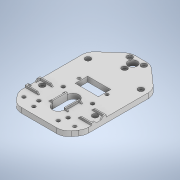
# Autodesk Inventor part: chassis
Saved by Autodesk Inventor 2020 (Build 240168000, 168)
## iProperties
Created: 2020-11-03
Part Number: chassis
Material: Generic
Document SubType Name: Modeling
Designer: alnwlsn
Density: 1 g/cm^3
Appearance: Default
Author: alnwlsn
Autodesk Inventor part; units mm, degrees
ref_plane "YZ Plane" through (0, 0, 0) normal (1, 0, 0) x (0, 1, 0)
ref_plane "XZ Plane" through (0, 0, 0) normal (0, 1, 0) x (-1, 0, 0)
sketch "Sketch1" plane through (0, 0, 0) normal (0, 1, 0) x (-1, 0, 0)
  line L0 (0, 0) -> (0, -80)
  line L1 (22.5, -100) -> (42.5, -100)
  line L2 (42.5, -100) -> (65, -80)
  line L3 (65, -80) -> (65, 0)
  line L4 (65, 0) -> (0, 0)
  line L5 (65, -80) -> (0, -80) construction
  line L6 (0, -80) -> (22.5, -100)
  line L7 (32.5, -100) -> (32.5, -80) construction
  line L8 (56, 0) -> (65, -12)
  line L9 (9, 0) -> (0, -12)
  dimension "d0" = 65
  dimension "d1" = 80
  dimension "d2" = 20
  dimension "d3" = 20
  dimension "d66" = 9
  dimension "d67" = 9
  dimension "d68" = 12
  dimension "d69" = 12
  constraints: 20 end point, 4 point on line, 3 perpendicular, 2 midpoint, 2 vertical, 1 parallel
  measures "d0" distance of L3.end L0.start
  measures "d1" distance of L2.end L3.end
  measures "d2" distance between parallel lines of L1 L5
  measures "d3" distance of L1.start L1.end
  measures "d66" distance of L3.end L8.start
  measures "d67" distance of L0.start L9.start
  measures "d68" distance of L0.start L9.end
  measures "d69" distance of L3.end L8.end
extrude "Extrusion1" add sketch "Sketch1" along normal blind 5 contours L9 L4 L8 L3 L2 L1 L6 L0
sketch "Sketch2" plane through (0, 5, 0) normal (0, 1, 0) x (1, 0, 0)
  line L0 (-1.2, 20) -> (-25.6, 20)
  line L1 (-25.6, 20) -> (-25.6, 32.2)
  line L2 (-25.6, 32.2) -> (-1.2, 32.2)
  line L3 (-1.2, 32.2) -> (-1.2, 20)
  line L4 (0, 33.4) -> (-26.8, 33.4)
  line L5 (-26.8, 33.4) -> (-26.8, 18.8)
  line L6 (-26.8, 18.8) -> (0, 18.8)
  line L7 (0, 18.8) -> (0, 33.4)
  line L8 (-56, 0) -> (0, 0) projected
  line L9 (-1.2, 23.8) -> (0, 23.8)
  line L10 (-1.2, 28.4) -> (0, 28.4)
  line L11 (0, 0) -> (0, 80) projected
  line L12 (-23.1, 18.8) -> (-23.1, 33.4)
  line L13 (-13.1, 18.8) -> (-13.1, 33.4)
  point P0 (-65, 0)
  point P1 (0, 28.4)
  point P2 (-13.1, 32.2)
  point P3 (-13.1, 20)
  point P4 (-23.1, 32.2)
  point P5 (-23.1, 20)
  dimension "d6" = 1.2
  dimension "d7" = 12.2
  dimension "d8" = 24.4
  dimension "d9" = 20
  dimension "d12" = 5
  dimension "d13" = 5
  dimension "d17" = 10
  dimension "d19" = 2.5
  constraints: 24 end point, 9 point on line, 6 perpendicular, 4 parallel, 1 horizontal, 3 other
  measures "d6" distance between parallel lines of L4 L2
  measures "d7" distance between parallel lines of L2 L0
  measures "d8" distance between parallel lines of L1 L3
  measures "d9" distance between parallel lines of L8 L0
  measures "d12" distance between parallel lines of L4 L10
  measures "d13" distance between parallel lines of L9 L6
  measures "d17" distance between parallel lines of L13 L12
  measures "d19" distance between parallel lines of L1 L12
extrude "Extrusion2" add sketch "Sketch2" along normal blind 2 contours L3 L9 L7 L6 L13 L0 | L12 L6 L5 L4 L2 L1 L0 | L13 L4 L7 L10 L3 L2
chamfer "Chamfer1" distance 2 angle 45 6 edges at (-0.6, 7, -23.8) (-0.6, 7, -28.4) (-13.1, 7, -19.4) (-23.1, 7, -19.4) (-23.1, 7, -32.8) (-13.1, 7, -32.8)
ref_plane "Work Plane1" through (-32.5, 0, 0) normal (1, 0, 0) x (0, 0, -1)
sketch "Sketch3" plane through (0, 5, 0) normal (0, 1, 0) x (1, 0, 0)
  line L0 (-25.1, 18.8) -> (-23.1, 18.8) projected
  line L1 (-13.1, 33.4) -> (0, 33.4) projected
  line L2 (-23.1, 18.8) -> (-13.1, 33.4) construction
  line L3 (-18.1, 26.1) -> (-18.1, 38.1) construction
  line L4 (-18.1, 26.1) -> (-18.1, 14.1) construction
  circle A0 centre (-18.1, 14.1) radius 1.7
  circle A1 centre (-18.1, 38.1) radius 1.7
  point P0 (0, 0)
  dimension "d20" = 24
  dimension "d21" = 3.4
  constraints: 6 end point, 2 centre point, 2 coincident, 1 collinear, 1 equal radius, 1 midpoint, 1 point on line, 1 vertical
  measures "d20" distance of L4.end L3.end
  measures "d21" diameter of A1
extrude "Extrusion3" cut sketch "Sketch3" against normal through all
mirror "Mirror1" about plane through (-32.5, 0, 0) normal (1, 0, 0) of "Extrusion2", "Extrusion3", "Chamfer1"
sketch "Sketch4" plane through (0, 0, 0) normal (0, -1, 0) x (1, 0, 0)
  line L0 (-22.5, -100) -> (-42.5, -100) projected
  line L1 (-32.5, -100) -> (-32.5, -92) construction
  circle A0 centre (-32.5, -92) radius 4.5
  line L2 (-42.2859, -97.6499) -> (-22.7141, -97.6499) construction
  line L3 (-42.2859, -97.6499) -> (-32.5, -80.7002) construction
  line L4 (-32.5, -80.7002) -> (-22.7141, -97.6499) construction
  line L5 (-37.3929, -89.1751) -> (-22.7141, -97.6499) construction
  circle A1 centre (-32.5, -84.0002) radius 1.65
  circle A2 centre (-25.572, -95.9999) radius 1.65
  circle A3 centre (-39.428, -95.9999) radius 1.65
  point P0 (0, 0)
  point P1 (-32.5, -97.6499)
  dimension "d24" = 9
  dimension "d25" = 13.856
  dimension "d26" = 3.3
  dimension "d27" = 8
  constraints: 10 end point, 6 tangent, 4 centre point, 3 midpoint, 2 equal length, 2 equal radius, 2 point on line, 1 coincident, 1 horizontal, 1 vertical
  measures "d24" diameter of A0
  measures "d25" distance of A2.centre A3.centre
  measures "d26" diameter of A2
  measures "d27" distance of L1.start L1.end
extrude "Extrusion4" cut sketch "Sketch4" against normal through all
sketch "Sketch5" plane through (0, 0, 0) normal (0, -1, 0) x (1, 0, 0)
  line L0 (-65, -80) -> (-65, -33.4) projected
  line L1 (-65, -53) -> (0, -53) construction
  line L2 (-56, 0) -> (0, 0) projected
  line L3 (-43.85, -46.9) -> (-21.15, -46.9)
  line L4 (-21.15, -46.9) -> (-21.15, -59.1)
  line L5 (-21.15, -59.1) -> (-43.85, -59.1)
  line L6 (-43.85, -59.1) -> (-43.85, -46.9)
  line L7 (-43.85, -46.9) -> (-21.15, -59.1) construction
  line L8 (-21.15, -46.9) -> (-43.85, -59.1) construction
  line L9 (0, 0) -> (0, -80) projected
  circle A0 centre (-46.25, -53) radius 1.5
  circle A1 centre (-18.75, -53) radius 1.5
  point P0 (-65, 0)
  point P1 (-32.5, -53)
  dimension "d30" = 53
  dimension "d31" = 22.7
  dimension "d32" = 12.2
  dimension "d33" = 13.75
  dimension "d34" = 13.75
  dimension "d35" = 3
  constraints: 14 end point, 4 point on line, 3 midpoint, 2 centre point, 2 horizontal, 2 parallel, 1 equal radius, 1 perpendicular
  measures "d30" distance between parallel lines of L1 L2
  measures "d31" distance between parallel lines of L4 L6
  measures "d32" distance between parallel lines of L3 L5
  measures "d33" distance of point (-32.5, -53) A1.centre
  measures "d34" distance of A0.centre point (-32.5, -53)
  measures "d35" diameter of A1
extrude "Extrusion5" cut sketch "Sketch5" against normal through all
sketch "Sketch6" plane through (0, 5, 0) normal (0, 1, 0) x (1, 0, 0)
  line L0 (-44.5, 6.75) -> (-20.5, 6.75) construction
  circle A0 centre (-44.5, 6.75) radius 1.65
  circle A1 centre (-20.5, 6.75) radius 1.65
  line L1 (-32.5, 6.75) -> (-32.5, 0) construction
  line L2 (-56, 0) -> (-9, 0) projected
  point P0 (-65, 0)
  dimension "d38" = 3.3
  dimension "d40" = 24
  constraints: 4 end point, 2 centre point, 2 coincident, 2 midpoint, 1 equal radius, 1 horizontal, 1 perpendicular
  measures "d38" diameter of A0
  measures "d40" distance of L0.start L0.end
extrude "Extrusion6" cut sketch "Sketch6" against normal through all
sketch "Sketch7" plane through (0, 5, 0) normal (0, 1, 0) x (1, 0, 0)
  line L0 (-32.5, 120) -> (-32.5, -20) projected
  line L1 (-57.5, 10) -> (-7.5, 10) construction
  line L2 (-56, 0) -> (0, 0) projected
  circle A0 centre (-57.5, 10) radius 1.65
  circle A1 centre (-7.5, 10) radius 1.65
  point P0 (-32.5, 10)
  point P1 (-65, 0)
  dimension "d43" = 10
  dimension "d44" = 3.3
  dimension "d45" = 50
  constraints: 2 centre point, 2 coincident, 2 end point, 1 equal radius, 1 horizontal, 1 midpoint, 1 point on line
  measures "d43" distance between parallel lines of L2 L1
  measures "d44" diameter of A0
  measures "d45" distance of L1.start L1.end
extrude "Extrusion7" cut sketch "Sketch7" against normal through all
sketch "Sketch8" plane through (0, 5, 0) normal (0, 1, 0) x (1, 0, 0)
  line L0 (-32.5, 120) -> (-32.5, -20) projected
  line L1 (-6.5, 74) -> (-58.5, 74) construction
  line L2 (-6.5, 29) -> (-58.5, 29) construction
  line L3 (-56, 0) -> (0, 0) projected
  circle A0 centre (-39.428, 95.9999) radius 1.65 projected
  circle A1 centre (-32.5, 84.0002) radius 1.65 projected
  circle A2 centre (-25.572, 95.9999) radius 1.65 projected
  point P0 (-32.5, 29)
  point P1 (-32.5, 74)
  point P2 (-65, 0)
  dimension "d48" = 45
  dimension "d49" = 52
  dimension "d50" = 29
  constraints: 7 coincident, 4 end point, 2 horizontal, 2 midpoint, 2 point on line, 1 parallel
  measures "d48" distance between parallel lines of L1 L2
  measures "d49" distance of L1.start L1.end
  measures "d50" distance from line of L3 L2.start
hole "Hole1" at (-6.5, 5, -74) at (-6.5, 5, -29) at (-58.5, 5, -29) at (-58.5, 5, -74) at (-32.5, 5, -84.0002) at (-39.428, 5, -95.9999) at (-25.572, 5, -95.9999) direction (0, -1, 0) diameter 3 end through all counterbore diameter 5.4 counterbore depth 2.3
fillet "Fillet1" radius 12 8 edges at (-65, 2.5, -12) (-56, 2.5, 0) (-65, 2.5, -80) (-42.5, 2.5, -100) (-22.5, 2.5, -100) (0, 2.5, -80) (0, 2.5, -12) (-9, 2.5, 0)
sketch "Sketch12" plane through (0, 5, 0) normal (0, 1, 0) x (1, 0, 0)
  arc A0 (-65, 16) -> (-62.6, 8.8) centre (-53, 16) ccw projected
  line L0 (-65, 18.8) -> (-65, 16) projected
  line L1 (-65, 18.8) -> (-65, 21.8) projected
  line L2 (-65, 23.8) -> (-65, 21.8) projected
  line L3 (-65, 28.4) -> (-65, 23.8) projected
  line L4 (-65, 30.4) -> (-65, 28.4) projected
  line L5 (-65, 30.4) -> (-65, 33.4) projected
  line L6 (-65, 74.6112) -> (-65, 33.4) projected
  arc A1 (-60.9724, 83.5801) -> (-65, 74.6112) centre (-53, 74.6112) ccw projected
  line L7 (-45.91, 96.9689) -> (-60.9724, 83.5801) projected
  arc A2 (-37.9376, 100) -> (-45.91, 96.9689) centre (-37.9376, 88) ccw projected
  line L8 (-27.0624, 100) -> (-37.9376, 100) projected
  arc A3 (-19.09, 96.9689) -> (-27.0624, 100) centre (-27.0624, 88) ccw projected
  line L9 (-4.0276, 83.5801) -> (-19.09, 96.9689) projected
  arc A4 (0, 74.6112) -> (-4.0276, 83.5801) centre (-12, 74.6112) ccw projected
  line L10 (0, 33.4) -> (0, 74.6112) projected
  line L11 (0, 30.4) -> (0, 33.4) projected
  line L12 (0, 28.4) -> (0, 30.4) projected
  line L13 (0, 23.8) -> (0, 28.4) projected
  line L14 (0, 21.8) -> (0, 23.8) projected
  line L15 (0, 18.8) -> (0, 21.8) projected
  line L16 (0, 16) -> (0, 18.8) projected
  arc A5 (-2.4, 8.8) -> (0, 16) centre (-12, 16) ccw projected
  line L17 (-5.4, 4.8) -> (-2.4, 8.8) projected
  arc A6 (-15, 0) -> (-5.4, 4.8) centre (-15, 12) ccw projected
  line L18 (-50, 0) -> (-15, 0) projected
  arc A7 (-59.6, 4.8) -> (-50, 0) centre (-50, 12) ccw projected
  line L19 (-62.6, 8.8) -> (-59.6, 4.8) projected
  line L20 (-62, 33.4) -> (-62, 30.4)
  line L21 (-62, 30.4) -> (-62, 28.4)
  line L22 (-62, 28.4) -> (-62, 23.8)
  line L23 (-62, 23.8) -> (-62, 21.8)
  line L24 (-62, 21.8) -> (-62, 18.8)
  line L25 (-62, 18.8) -> (-62, 16)
  arc A8 (-62, 16) -> (-60.2, 10.6) centre (-53, 16) ccw
  line L26 (-60.2, 10.6) -> (-57.2, 6.6)
  arc A9 (-57.2, 6.6) -> (-50, 3) centre (-50, 12) ccw
  line L27 (-50, 3) -> (-15, 3)
  arc A10 (-15, 3) -> (-7.8, 6.6) centre (-15, 12) ccw
  line L28 (-7.8, 6.6) -> (-4.8, 10.6)
  arc A11 (-4.8, 10.6) -> (-3, 16) centre (-12, 16) ccw
  line L29 (-3, 16) -> (-3, 18.8)
  line L30 (-3, 18.8) -> (-3, 21.8)
  line L31 (-3, 21.8) -> (-3, 23.8)
  line L32 (-3, 23.8) -> (-3, 28.4)
  line L33 (-3, 28.4) -> (-3, 30.4)
  line L34 (-3, 30.4) -> (-3, 33.4)
  line L35 (-3, 33.4) -> (-3, 74.6112)
  arc A12 (-3, 74.6112) -> (-6.0207, 81.3379) centre (-12, 74.6112) ccw
  line L36 (-6.0207, 81.3379) -> (-21.0831, 94.7267)
  arc A13 (-21.0831, 94.7267) -> (-27.0624, 97) centre (-27.0624, 88) ccw
  line L37 (-27.0624, 97) -> (-37.9376, 97)
  arc A14 (-37.9376, 97) -> (-43.9169, 94.7267) centre (-37.9376, 88) ccw
  line L38 (-43.9169, 94.7267) -> (-58.9793, 81.3379)
  arc A15 (-58.9793, 81.3379) -> (-62, 74.6112) centre (-53, 74.6112) ccw
  line L39 (-62, 74.6112) -> (-62, 33.4)
  arc A16 (-15, 0) -> (-5.4, 4.8) centre (-15, 12) ccw projected
  line L40 (-5.4, 4.8) -> (-2.4, 8.8) projected
  arc A17 (-2.4, 8.8) -> (0, 16) centre (-12, 16) ccw projected
  line L41 (0, 16) -> (0, 18.8) projected
  line L42 (0, 18.8) -> (-13.1, 18.8) projected
  line L43 (-13.1, 18.8) -> (-13.1, 20) projected
  line L44 (-13.1, 20) -> (-1.2, 20) projected
  line L45 (-1.2, 20) -> (-1.2, 23.8) projected
  line L46 (-1.2, 23.8) -> (0, 23.8) projected
  line L47 (0, 23.8) -> (0, 28.4) projected
  line L48 (0, 28.4) -> (-1.2, 28.4) projected
  line L49 (-1.2, 28.4) -> (-1.2, 32.2) projected
  line L50 (-1.2, 32.2) -> (-13.1, 32.2) projected
  line L51 (-13.1, 32.2) -> (-13.1, 33.4) projected
  line L52 (-13.1, 33.4) -> (0, 33.4) projected
  line L53 (0, 33.4) -> (0, 74.6112) projected
  arc A18 (0, 74.6112) -> (-4.0276, 83.5801) centre (-12, 74.6112) ccw projected
  line L54 (-4.0276, 83.5801) -> (-19.09, 96.9689) projected
  arc A19 (-19.09, 96.9689) -> (-27.0624, 100) centre (-27.0624, 88) ccw projected
  line L55 (-27.0624, 100) -> (-37.9376, 100) projected
  arc A20 (-37.9376, 100) -> (-45.91, 96.9689) centre (-37.9376, 88) ccw projected
  line L56 (-45.91, 96.9689) -> (-60.9724, 83.5801) projected
  arc A21 (-60.9724, 83.5801) -> (-65, 74.6112) centre (-53, 74.6112) ccw projected
  line L57 (-65, 74.6112) -> (-65, 33.4) projected
  line L58 (-65, 33.4) -> (-51.9, 33.4) projected
  line L59 (-51.9, 33.4) -> (-51.9, 32.2) projected
  line L60 (-51.9, 32.2) -> (-63.8, 32.2) projected
  line L61 (-63.8, 32.2) -> (-63.8, 28.4) projected
  line L62 (-63.8, 28.4) -> (-65, 28.4) projected
  line L63 (-65, 28.4) -> (-65, 23.8) projected
  line L64 (-65, 23.8) -> (-63.8, 23.8) projected
  line L65 (-63.8, 23.8) -> (-63.8, 20) projected
  line L66 (-63.8, 20) -> (-51.9, 20) projected
  line L67 (-51.9, 20) -> (-51.9, 18.8) projected
  line L68 (-51.9, 18.8) -> (-65, 18.8) projected
  line L69 (-65, 18.8) -> (-65, 16) projected
  arc A22 (-65, 16) -> (-62.6, 8.8) centre (-53, 16) ccw projected
  line L70 (-62.6, 8.8) -> (-59.6, 4.8) projected
  arc A23 (-59.6, 4.8) -> (-50, 0) centre (-50, 12) ccw projected
  line L71 (-50, 0) -> (-15, 0) projected
  line L72 (-39.4, 20) -> (-39.4, 32.2) projected
  line L73 (-39.4, 32.2) -> (-41.9, 32.2) projected
  line L74 (-41.9, 32.2) -> (-41.9, 33.4) projected
  line L75 (-41.9, 33.4) -> (-38.2, 33.4) projected
  line L76 (-38.2, 33.4) -> (-38.2, 18.8) projected
  line L77 (-38.2, 18.8) -> (-41.9, 18.8) projected
  line L78 (-41.9, 18.8) -> (-41.9, 20) projected
  line L79 (-41.9, 20) -> (-39.4, 20) projected
  circle A24 centre (-18.1, 38.1) radius 1.7 projected
  circle A25 centre (-18.1, 14.1) radius 1.7 projected
  line L80 (-25.6, 32.2) -> (-25.6, 20) projected
  line L81 (-25.6, 20) -> (-23.1, 20) projected
  line L82 (-23.1, 20) -> (-23.1, 18.8) projected
  line L83 (-23.1, 18.8) -> (-26.8, 18.8) projected
  line L84 (-26.8, 18.8) -> (-26.8, 33.4) projected
  line L85 (-26.8, 33.4) -> (-23.1, 33.4) projected
  line L86 (-23.1, 33.4) -> (-23.1, 32.2) projected
  line L87 (-23.1, 32.2) -> (-25.6, 32.2) projected
  circle A26 centre (-46.9, 14.1) radius 1.7 projected
  circle A27 centre (-46.9, 38.1) radius 1.7 projected
  circle A28 centre (-32.5, 92) radius 4.5 projected
  circle A29 centre (-18.75, 53) radius 1.5 projected
  line L88 (-21.15, 46.9) -> (-43.85, 46.9) projected
  line L89 (-43.85, 46.9) -> (-43.85, 59.1) projected
  line L90 (-43.85, 59.1) -> (-21.15, 59.1) projected
  line L91 (-21.15, 59.1) -> (-21.15, 46.9) projected
  circle A30 centre (-46.25, 53) radius 1.5 projected
  circle A31 centre (-44.5, 6.75) radius 1.65 projected
  circle A32 centre (-20.5, 6.75) radius 1.65 projected
  circle A33 centre (-57.5, 10) radius 1.65 projected
  circle A34 centre (-7.5, 10) radius 1.65 projected
  circle A35 centre (-25.572, 95.9999) radius 2.7 projected
  circle A36 centre (-32.5, 84.0002) radius 2.7 projected
  circle A37 centre (-58.5, 29) radius 2.7 projected
  circle A38 centre (-6.5, 74) radius 2.7 projected
  circle A39 centre (-6.5, 29) radius 2.7 projected
  circle A40 centre (-58.5, 74) radius 2.7 projected
  circle A41 centre (-39.428, 95.9999) radius 2.7 projected
  line L92 (-9.7823, 43.7283) -> (-9.7823, 63.7283) construction
  line L93 (-3.4383, 43.7283) -> (-3.4383, 63.7283)
  line L94 (-16.1263, 63.7283) -> (-16.1263, 43.7283)
  arc A42 (-16.1263, 43.7283) -> (-3.4383, 43.7283) centre (-9.7823, 43.7283) ccw
  arc A43 (-3.4383, 63.7283) -> (-16.1263, 63.7283) centre (-9.7823, 63.7283) ccw
  line L95 (-32.5, 0) -> (-32.5, 100)
  circle A44 centre (-32.5, 84.0002) radius 4.5
  line L96 (-32.5, 75.0002) -> (-18.8145, 98.7043)
  line L97 (-32.5, 75.0002) -> (-47.7486, 101.4116)
  circle A45 centre (-39.428, 95.9999) radius 4.5 construction
  line L98 (-32.5, 13) -> (-32.5, 36.9) construction
  line L99 (-38, 13) -> (-38, 36.9)
  line L100 (-27, 36.9) -> (-27, 13)
  arc A46 (-38, 13) -> (-27, 13) centre (-32.5, 13) ccw
  arc A47 (-27, 36.9) -> (-38, 36.9) centre (-32.5, 36.9) ccw
  circle A48 centre (-27.5, 64.6863) radius 3
  circle A49 centre (-20.3437, 90.0556) radius 3
  circle A50 centre (-11.1883, 81.9174) radius 3
  circle A51 centre (-27.5, 77.6605) radius 3
  line L101 (-25.3214, 62.6239) -> (-9.0097, 79.855)
  line L102 (-30.5, 64.6863) -> (-30.5, 77.6605)
  line L103 (-61.5617, 43.7283) -> (-61.5617, 63.7283)
  line L104 (-48.8737, 63.7283) -> (-48.8737, 43.7283)
  arc A52 (-61.5617, 43.7283) -> (-48.8737, 43.7283) centre (-55.2177, 43.7283) ccw
  arc A53 (-48.8737, 63.7283) -> (-61.5617, 63.7283) centre (-55.2177, 63.7283) ccw
  circle A54 centre (-37.5, 64.6863) radius 3
  circle A55 centre (-44.6563, 90.0556) radius 3
  circle A56 centre (-53.8117, 81.9174) radius 3
  circle A57 centre (-37.5, 77.6605) radius 3
  line L105 (-39.6786, 62.6239) -> (-55.9903, 79.855)
  line L106 (-34.5, 64.6863) -> (-34.5, 77.6605)
  line L107 (-18.0582, 22.7364) -> (-18.0582, 30.5446) construction
  line L108 (-21.9699, 22.7364) -> (-21.9699, 30.5446)
  line L109 (-14.1465, 30.5446) -> (-14.1465, 22.7364)
  arc A58 (-21.9699, 22.7364) -> (-14.1465, 22.7364) centre (-18.0582, 22.7364) ccw
  arc A59 (-14.1465, 30.5446) -> (-21.9699, 30.5446) centre (-18.0582, 30.5446) ccw
  line L110 (-43.0301, 22.7364) -> (-43.0301, 30.5446)
  line L111 (-50.8535, 30.5446) -> (-50.8535, 22.7364)
  arc A60 (-50.8535, 22.7364) -> (-43.0301, 22.7364) centre (-46.9418, 22.7364) ccw
  arc A61 (-43.0301, 30.5446) -> (-50.8535, 30.5446) centre (-46.9418, 30.5446) ccw
  line L112 (-46.6077, 6.8915) -> (-50.8118, 6.8915) construction
  line L113 (-46.6077, 3.3915) -> (-50.8118, 3.3915)
  line L114 (-50.8118, 10.3915) -> (-46.6077, 10.3915)
  arc A62 (-46.6077, 3.3915) -> (-46.6077, 10.3915) centre (-46.6077, 6.8915) ccw
  arc A63 (-50.8118, 10.3915) -> (-50.8118, 3.3915) centre (-50.8118, 6.8915) ccw
  line L115 (-18.3923, 3.3915) -> (-14.1882, 3.3915)
  line L116 (-14.1882, 10.3915) -> (-18.3923, 10.3915)
  arc A64 (-18.3923, 10.3915) -> (-18.3923, 3.3915) centre (-18.3923, 6.8915) ccw
  arc A65 (-14.1882, 3.3915) -> (-14.1882, 10.3915) centre (-14.1882, 6.8915) ccw
  point P0 (0, 0)
  point P1 (-9.7823, 53.7283)
  point P2 (-32.5, 24.95)
  point P3 (-30.0981, 79.1605)
  point P4 (-9.1952, 84.1597)
  point P5 (-18.3506, 92.2978)
  point P6 (-22.9418, 91.5556)
  point P7 (-55.8048, 84.1597)
  point P8 (-34.9019, 79.1605)
  point P9 (-42.0582, 91.5556)
  point P10 (-46.6494, 92.2978)
  point P11 (-18.0582, 26.6405)
  point P12 (-48.7097, 6.8915)
  dimension "d78" = 6
  dimension "d72" = 3
  dimension "d73" = 9
  dimension "d74" = 11
  dimension "d75" = 10
  dimension "d76" = 10
  dimension "d77" = 20
  dimension "d79" = 5
  dimension "d80" = 5
  constraints: 98 end point, 48 point on circle, 28 centre point, 26 symmetric about line, 23 tangent, 6 midpoint, 5 vertical, 4 parallel, 3 point on line, 2 coincident, 2 equal radius, 1 horizontal, 52 other
  measures "d72" distance between parallel lines of L6 L39
  measures "d73" diameter of A44
  measures "d74" distance between parallel lines of L100 L99
  measures "d75" distance from line of L88 L99.end
  measures "d76" distance from line of L27 L99.start
  measures "d77" distance of L92.start L92.end
  measures "d79" distance from line of L95 point (-27.5, 77.66)
  measures "d80" distance from line of L95 A48.centre
extrude "Extrusion8" [suppressed]
sketch "Sketch13" plane through (0, 5, 0) normal (0, 1, 0) x (1, 0, 0)
  line L0 (-38.2, 33.4) -> (-38.2, 18.8) projected
  line L1 (-26.8, 33.4) -> (-26.8, 18.8) projected
  line L2 (-32.5, 18.8) -> (-32.5, 33.4) construction
  line L3 (-26.8, 18.8) -> (-26.8, 33.4)
  line L4 (-38.2, 33.4) -> (-38.2, 18.8)
  arc A0 (-38.2, 18.8) -> (-26.8, 18.8) centre (-32.5, 18.8) ccw
  arc A1 (-26.8, 33.4) -> (-38.2, 33.4) centre (-32.5, 33.4) ccw
  point P0 (0, 0)
  point P1 (-32.5, 26.1)
  constraints: 8 end point, 4 point on circle, 4 tangent, 2 centre point, 1 midpoint, 1 parallel, 1 vertical
extrude "Extrusion9" cut sketch "Sketch13" against normal through all
equation "\"d67\" = d66"
equation "\"d69\" = d68"
equation "\"d13\" = d12"
equation "\"d34\" = d33"
body "Solid1"
